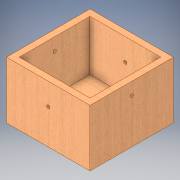
# Autodesk Inventor part: Box
Saved by Autodesk Inventor 2017 (Build 210142000, 142)
## iProperties
Created: 2017-01-25
Part Number: Box
Material: Wood (Cherry)
Document SubType Name: Modeling
Designer: aribu
Density: 0.63 g/cm^3
Appearance: Cherry - Natural Low Gloss
Author: aribu
Autodesk Inventor part; units mm, degrees
ref_plane "YZ Plane" through (0, 0, 0) normal (1, 0, 0) x (0, 1, 0)
ref_plane "XZ Plane" through (0, 0, 0) normal (0, 1, 0) x (-1, 0, 0)
ref_plane "XY Plane" through (0, 0, 0) normal (0, 0, 1) x (1, 0, 0)
sketch "Sketch1" plane through (0, 0, 0) normal (0, 1, 0) x (-1, 0, 0)
  line L0 (66.7958, 75.9213) -> (-75.4442, 75.9213)
  line L1 (-75.4442, 75.9213) -> (-75.4442, -66.3187)
  line L2 (-75.4442, -66.3187) -> (66.7958, -66.3187)
  line L3 (66.7958, -66.3187) -> (66.7958, 75.9213)
  line L4 (79.4958, 88.6213) -> (-88.1442, 88.6213)
  line L5 (-88.1442, 88.6213) -> (-88.1442, -79.0187)
  line L6 (-88.1442, -79.0187) -> (79.4958, -79.0187)
  line L7 (79.4958, -79.0187) -> (79.4958, 88.6213)
  point P0 (0, 0)
  dimension "d0" = 142.24
  dimension "d1" = 142.24
  dimension "d2" = 12.7
  dimension "d3" = 12.7
  dimension "d4" = 12.7
  dimension "d5" = 12.7
  constraints: 16 end point, 4 parallel, 2 horizontal, 2 perpendicular
  measures "d0" distance of L0.start L0.end
  measures "d1" distance of L2.end L0.start
  measures "d2" distance between parallel lines of L3 L7
  measures "d3" distance between parallel lines of L1 L5
  measures "d4" distance between parallel lines of L6 L2
  measures "d5" distance between parallel lines of L4 L0
extrude "Extrusion1" add sketch "Sketch1" along normal blind 101.6
sketch "Sketch2" plane through (0, 0, 0) normal (0, -1, 0) x (1, 0, 0)
  line L0 (-79.4958, 88.6213) -> (88.1442, 88.6213) projected
  line L1 (-79.4958, -79.0187) -> (-79.4958, 88.6213) projected
  line L2 (88.1442, 88.6213) -> (-79.4958, 88.6213)
  line L3 (-79.4958, 88.6213) -> (-79.4958, -79.0187)
  line L4 (-79.4958, -79.0187) -> (88.1442, -79.0187)
  line L5 (88.1442, -79.0187) -> (88.1442, 88.6213)
  point P0 (0, 0)
  constraints: 8 end point, 2 parallel, 1 horizontal, 1 perpendicular
extrude "Extrusion2" add sketch "Sketch2" along normal blind 12.7
sketch "Sketch3" plane through (88.1442, 101.6, 88.6213) normal (1, 0, 0) x (0, 0, -1)
  circle A0 centre (83.82, -25.4) radius 3.175
  line L0 (0, 0) -> (167.64, 0) projected
  line L1 (0, -114.3) -> (0, 0) projected
  point P0 (88.6213, -101.6)
  dimension "d10" = 6.35
  dimension "d11" = 25.4
  dimension "d12" = 83.82
  constraints: 1 centre point
  measures "d10" diameter of A0
  measures "d11" distance from line of A0.centre L0
  measures "d12" distance from line of L1 A0.centre
extrude "Extrusion3" cut sketch "Sketch3" against normal blind 177.8
sketch "Sketch4" plane through (-79.4958, 101.6, 88.6213) normal (0, 0, 1) x (1, 0, 0)
  circle A0 centre (83.82, -44.45) radius 3.175
  line L0 (0, 0) -> (167.64, 0) projected
  line L1 (0, 0) -> (0, -114.3) projected
  point P0 (79.4958, -101.6)
  dimension "d15" = 6.35
  dimension "d16" = 44.45
  dimension "d17" = 83.82
  constraints: 1 centre point
  measures "d15" diameter of A0
  measures "d16" distance from line of A0.centre L0
  measures "d17" distance from line of A0.centre L1
extrude "Extrusion4" cut sketch "Sketch4" against normal blind 177.8
body "Solid1"
